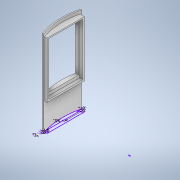
# Autodesk Inventor part: face_v3
Saved by Autodesk Inventor 2022 (Build 260153000, 153)
## iProperties
Created: 2023-04-03
Part Number: face_v3
Material: Generic
Document SubType Name: Modeling
Designer: emp
Density: 1 g/cm^3
Appearance: Default
Author: emp
Autodesk Inventor part; units mm, degrees
ref_plane "YZ Plane" through (0, 0, 0) normal (1, 0, 0) x (0, 1, 0)
ref_plane "XZ Plane" through (0, 0, 0) normal (0, 1, 0) x (-1, 0, 0)
ref_plane "XY Plane" through (0, 0, 0) normal (0, 0, 1) x (1, 0, 0)
sketch "Sketch1" plane through (0, 0, 0) normal (0, 1, 0) x (-1, 0, 0)
  line L0 (0, 0) -> (2, 0) construction
  line L1 (0, -75) -> (2, -75) construction
  line L2 (0, -73) -> (2.4733, -73)
  line L3 (1.3383, -13) -> (1.3383, -5.3327) construction
  line L4 (6.5938, -37.5) -> (0, -37.5) construction
  line L5 (2.0086, -8.9832) -> (-0.0001, -8.9832) construction
  arc A0 (0.4733, -73) -> (-2.5001, -8.9832) centre (-105.0089, -45.8218) ccw
  arc A1 (2.4733, -73) -> (-0.5001, -8.9832) centre (-103.0089, -45.8218) ccw
  line L6 (-0.5001, -8.9832) -> (-2.5001, -8.9832)
  line L7 (-0.9649, -13.5728) -> (-5.9649, -13.5728)
  line L8 (-5.9649, -13.5728) -> (-5.9649, -10.8228)
  line L9 (-5.9649, -10.8228) -> (-1.8575, -10.8228)
  line L10 (-3.6617, -68.25) -> (-8.7098, -68.25) construction
  line L11 (1.5844, -68.25) -> (-5.9649, -68.25)
  line L12 (-5.9649, -68.25) -> (-5.9649, -71)
  line L13 (-5.9649, -71) -> (0.9685, -71)
  line L14 (-5.9649, -13.5728) -> (-5.9649, -68.25)
  line L15 (-0.9649, -13.5728) -> (-0.9649, -15.2728)
  line L16 (-0.9649, -66.55) -> (1.9279, -66.55)
  line L17 (3.9279, -66.55) -> (1.9279, -66.55)
  line L18 (-0.9649, -15.2728) -> (-0.4532, -15.2728)
  line L19 (1.5468, -15.2728) -> (-0.4532, -15.2728)
  line L20 (-0.9649, -15.2728) -> (-0.9649, -66.55)
  line L21 (-0.9649, -66.55) -> (-0.9649, -68.25)
  point P0 (0.0167, -6.9833)
  point P1 (2, 0)
  point P2 (4.5938, -37.5)
  point P3 (0, -41)
  point P4 (0, -15)
  point P5 (0, -67.5)
  point P6 (0, -69)
  point P7 (0, -13)
  point P8 (3.8363, -67.0175)
  point P9 (-3.6617, -13.5728)
  point P10 (0.9193, -71)
  point P11 (1.5637, -68.25)
  point P12 (2.3337, -10.8228)
  point P13 (-3.6617, -10.8228)
  point P14 (1.3383, -13.5728)
  point P15 (3.6, -37.5)
  point P16 (5.6, -37.5)
  point P17 (-0.5333, -15)
  point P18 (1.4667, -15)
  dimension "d1" = 2
  dimension "d3" = 2
  dimension "d4" = 2
  dimension "d5" = 2
  dimension "d6" = 32
  dimension "d8" = 3.6
  dimension "d9" = 2
  dimension "d10" = 2.5
  dimension "d11" = 2
  dimension "d12" = 5
  dimension "d29" = 1.7
  constraints: 44 end point, 8 point on line, 7 horizontal, 7 point on circle, 4 perpendicular, 3 coincident, 3 collinear, 2 vertical, 1 centre point, 12 other
  measures "d1" distance of L0.start L0.end
  measures "d3" distance of L1.start L1.end
  measures "d4" distance of point (0, -75) L2.start
  measures "d5" distance of L5.end point (0.017, -6.983)
  measures "d6" distance of L2.start point (0, -41)
  measures "d8" distance of point (3.6, -37.5) L4.end
  measures "d9" distance of point (3.6, -37.5) point (5.6, -37.5)
  measures "d10" distance of L5.end L6.end
  measures "d11" distance of L6.end L6.start
  measures "d12" distance of L7.start L7.end
  measures "d29" distance of L7.start L15.end
extrude "Extrusion12" add sketch "Sketch1" along normal blind 138 contours A0 L17 A1 L2 | L17 A0 L19 A1 | L19 A0 L6 A1
extrude "Extrusion13" add sketch "Sketch1" along normal blind 133 contours L13 L12 L11 A0 | L11 L21 L16 A0 | L16 L20 L18 A0 | L11 L14 L7 L15 L20 L21 | L18 L15 A0 | L8 L9 A0 L7
extrude "Extrusion14" cut sketch "Sketch1" along normal blind 129 contours L17 A0 L19 A1
extrude "Extrusion15" cut sketch "Sketch1" along normal blind 131 contours L11 L14 L7 L15 L20 L21
extrude "Extrusion16" cut sketch "Sketch1" along normal blind 129 contours L16 L20 L18 A0
extrude "Extrusion17" add sketch "Sketch1" along normal blind 51 contours L17 A0 L19 A1 | L16 L20 L18 A0
extrude "Extrusion18" add sketch "Sketch1" along normal blind 46 contours L11 L14 L7 L15 L20 L21
extrude "Extrusion20" cut sketch "Sketch1" along normal blind 43 contours L13 L12 L11 A0 | L11 L21 L16 A0 | L16 L20 L18 A0 | L11 L14 L7 L15 L20 L21 | L18 L15 A0 | L8 L9 A0 L7
body "Solid2"
